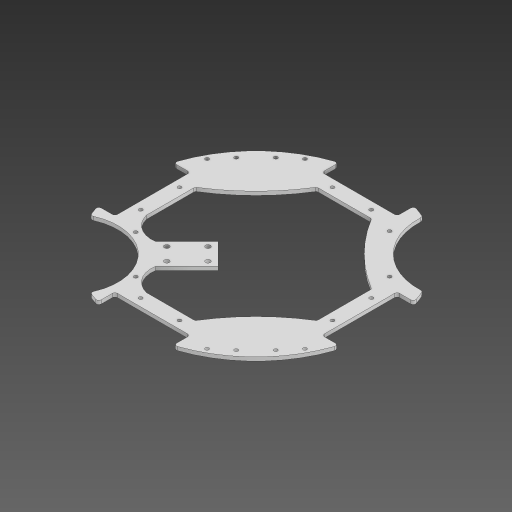
# Autodesk Inventor part: bottom
Saved by Autodesk Inventor 2023 (Build 270158000, 158)
## iProperties
Created: 2025-06-24
Part Number: bottom
Material: Типовые
Document SubType Name: Modeling
Designer: daa
Density: 1 g/cm^3
Appearance: По умолчанию
Author: daa
Autodesk Inventor part; units mm, degrees
ref_plane "YZ Plane" through (0, 0, 0) normal (1, 0, 0) x (0, 1, 0)
ref_plane "XZ Plane" through (0, 0, 0) normal (0, 1, 0) x (-1, 0, 0)
ref_plane "XY Plane" through (0, 0, 0) normal (0, 0, 1) x (1, 0, 0)
sketch "Эскиз1" plane through (0, 0, 0) normal (0, 1, 0) x (-1, 0, 0)
  line L0 (-79, -47.2724) -> (-79, 14.7276)
  line L1 (91.5447, -47.2724) -> (91.5447, 14.7276)
  line L2 (-79, -47.2724) -> (-93, -47.2724)
  line L3 (-79, 14.7276) -> (-93, 14.7276)
  line L4 (91.5447, -47.2724) -> (105.5447, -47.2724)
  line L5 (91.5447, 14.7276) -> (105.5447, 14.7276)
  line L6 (-24.7276, -101.5447) -> (37.2724, -101.5447)
  line L7 (-24.7276, 69) -> (37.2724, 69)
  line L8 (-24.7276, 69) -> (-24.7276, 83)
  line L9 (37.2724, 69) -> (37.2724, 83)
  line L10 (37.2724, -101.5447) -> (37.2724, -115.5447)
  line L11 (-24.7276, -101.5447) -> (-24.7276, -115.5447)
  arc A0 (-93, -47.2724) -> (-24.7276, -115.5447) centre (6.2724, -16.2724) ccw
  arc A1 (105.5447, 14.7276) -> (37.2724, 83) centre (6.2724, -16.2724) ccw
  arc A2 (-24.7276, 83) -> (-93, 14.7276) centre (6.2724, -16.2724) ccw
  arc A3 (37.2724, -115.5447) -> (105.5447, -47.2724) centre (6.2724, -16.2724) ccw
  dimension "d29" = 62
  dimension "d31" = 62
  dimension "d33" = 14
  dimension "d34" = 14
  dimension "d35" = 62
  dimension "d36" = 62
  dimension "d39" = 14
  dimension "d40" = 14
  constraints: 24 end point, 8 point on circle, 4 centre point, 4 horizontal, 3 parallel, 3 vertical, 2 point on line, 1 concentric
  measures "d29" distance of L0.start L0.end
  measures "d31" distance of L1.start L1.end
  measures "d33" distance of L0.end L3.end
  measures "d34" distance of L1.end L5.end
  measures "d35" distance of L6.start L6.end
  measures "d36" distance of L7.start L7.end
  measures "d39" distance of L7.start L8.end
  measures "d40" distance of L6.start L11.end
extrude "motor" add sketch "Эскиз1" along normal blind 3
sketch "Эскиз2" plane through (0, 3, 0) normal (0, 1, 0) x (1, 0, 0)
  arc A0 (24.7276, -83) -> (93, -14.7276) centre (-6.2724, 16.2724) ccw projected
  arc A1 (-37.2724, 115.5447) -> (-105.5447, 47.2724) centre (-6.2724, 16.2724) ccw projected
  circle A2 centre (-6.2724, 16.2724) radius 104
  line L0 (-6.2724, 16.2724) -> (-6.2724, -50.7276)
  arc A3 (-37.2724, 115.5447) -> (-105.5447, 47.2724) centre (-6.2724, 16.2724) ccw projected
  line L1 (-80.4681, -6.5111) -> (-32.5193, -54.4602)
  line L2 (-101.8495, -24.7276) -> (-47.2724, -79.3051)
  arc A4 (-105.5447, -14.7276) -> (-37.2724, -83) centre (-6.2724, 16.2724) ccw projected
  arc A5 (-47.2724, -79.3051) -> (-101.8495, -24.7276) centre (-83.4673, -60.9227) ccw
  arc A6 (24.7276, -83) -> (93, -14.7276) centre (-6.2724, 16.2724) ccw projected
  line L3 (24.3063, 98.7917) -> (72.2554, 50.8426)
  line L4 (35.8032, 111.3809) -> (88.8362, 58.3479)
  arc A7 (93, 47.2724) -> (24.7276, 115.5447) centre (-6.2724, 16.2724) ccw
  arc A8 (35.8032, 111.3809) -> (88.8362, 58.3479) centre (85.4903, 108.035) ccw
  line L5 (-91.5447, -14.7276) -> (-105.5447, -14.7276) projected
  line L6 (-105.5447, -14.7276) -> (-80, -14.7276)
  point P0 (0, 0)
  point P1 (-6.2724, -50.7276)
  point P2 (-101.8495, -24.7276)
  point P3 (-47.2722, -79.3049)
  dimension "d181" = 208
  dimension "d190" = 67
  dimension "d205" = 77.184
  dimension "d207" = 28
  dimension "d208" = 10
  dimension "d214" = 10
  constraints: 12 end point, 7 point on circle, 4 centre point, 2 tangent, 1 point on line, 1 vertical
  measures "d181" diameter of A2
  measures "d190" distance of L0.end L0.start
  measures "d205" distance of L2.start L2.end
  measures "d207" distance between parallel lines of L1 L2
  measures "d208" horizontal distance of A2.end L2.end
  measures "d214" vertical distance of L2.start L5.end
extrude "ball" cut sketch "Эскиз2" against normal blind 3 contours A2 L2 | L2 A5 | L4 A2 | A8 L4
sketch "Эскиз3" plane through (0, 3, 0) normal (0, 1, 0) x (1, 0, 0)
  arc A0 (93, 47.2724) -> (24.7276, 115.5447) centre (-6.2724, 16.2724) ccw projected
  line L0 (-6.2724, 16.2724) -> (97.7276, 16.2724) construction
  line L1 (67.2668, 89.8115) -> (-62.5447, -40)
  circle A1 centre (70.5306, -44.2673) radius 1.5
  circle A2 centre (54.2672, -60.5308) radius 1.5
  circle A3 centre (41.3053, -71.6104) radius 1.5
  circle A4 centre (81.6104, -31.3053) radius 1.5
  arc A5 (24.7276, -83) -> (93, -14.7276) centre (-6.2724, 16.2724) ccw projected
  line L2 (-6.2724, 16.2724) -> (97.7276, 16.2724) construction
  line L3 (-79.8115, 89.8115) -> (67.2668, -57.2668)
  line L4 (-91.5447, 47.2724) -> (-91.5447, -14.7276) projected
  line L5 (-91.5447, 16.2724) -> (79, 16.2724)
  line L6 (24.7276, 101.5447) -> (-37.2724, 101.5447) projected
  line L7 (-6.2724, 101.5447) -> (-6.2724, -69)
  line L8 (-6.2724, 101.5447) -> (-6.2724, -69)
  line L9 (-91.5447, 47.2724) -> (-91.5447, -14.7276) projected
  arc A6 (24.7276, -83) -> (93, -14.7276) centre (-6.2724, 16.2724) ccw projected
  circle A7 centre (-66.812, 93.0753) radius 1.5
  circle A8 centre (-83.0755, 76.8119) radius 1.5
  circle A9 centre (-94.1551, 63.85) radius 1.5
  circle A10 centre (-53.85, 104.1551) radius 1.5
  point P0 (0, 0)
  point P1 (67.2668, -57.2668)
  point P2 (67.2668, -57.2668)
  point P3 (-105.5447, 47.2724)
  point P4 (-79.8115, 89.8115)
  point P5 (-79.8115, 89.8115)
  point P6 (-79.8115, 89.8115)
  dimension "d65" = 3
  dimension "d66" = 3
  dimension "d67" = 3
  dimension "d68" = 3
  dimension "d69" = 23
  dimension "d71" = 57
  dimension "d74" = -12.962
  dimension "d78" = 25.9614
  constraints: 14 end point, 8 centre point, 8 symmetric about line, 4 point on circle, 3 midpoint, 2 horizontal, 2 vertical, 1 point on line, 4 other
  measures "d65" diameter of A1
  measures "d66" diameter of A2
  measures "d67" diameter of A3
  measures "d68" diameter of A4
  measures "d69" distance of A2.centre A1.centre
  measures "d71" distance of A3.centre A4.centre
  measures "d74" vertical distance of A1.centre A4.centre
  measures "d78" vertical distance of A4.centre point (67.267, -57.267)
extrude "hand_mount" cut sketch "Эскиз3" against normal blind 10
sketch "Эскиз4" plane through (0, 3, 0) normal (0, 1, 0) x (1, 0, 0)
  circle A0 centre (-6.2724, 16.2724) radius 104
  arc A1 (-37.2724, 115.5447) -> (-105.5447, 47.2724) centre (-6.2724, 16.2724) ccw projected
  line L0 (-37.2724, -69) -> (24.7276, -69) projected
  line L1 (-79.0447, -1.2276) -> (-79.0447, 38.7724)
  line L2 (-91.5447, 47.2724) -> (-91.5447, -14.7276) projected
  line L3 (-37.2724, -69) -> (24.7276, -69) projected
  line L4 (24.7276, 101.5447) -> (-37.2724, 101.5447) projected
  line L5 (66.5, -6.2276) -> (66.5, 38.7724)
  line L6 (-23.7724, -56.5) -> (16.2276, -56.5)
  line L7 (-28.7724, 89.0447) -> (16.2276, 89.0447)
  arc A2 (16.2276, 89.0447) -> (66.5, 38.7724) centre (144.4083, 166.953) ccw
  arc A3 (66.5, -6.2276) -> (16.2276, -56.5) centre (148.0441, -138.0441) ccw
  arc A4 (-79.0447, 38.7724) -> (-28.7724, 89.0447) centre (-160.5888, 170.5888) ccw
  line L8 (-30.6674, 9.5549) -> (-12.9897, -8.1229)
  line L9 (-12.9897, -8.1229) -> (-38.7992, -33.9322)
  line L10 (-38.7992, -33.9322) -> (-56.4768, -16.2545)
  line L11 (-56.4768, -16.2545) -> (-30.6674, 9.5549)
  circle A5 centre (-31.3151, 1.7173) radius 2
  circle A6 centre (-20.8273, -8.7706) radius 2
  circle A7 centre (-48.273, -15.2405) radius 2
  circle A8 centre (-37.7852, -25.7283) radius 2
  arc A9 (-79.0447, -1.2276) -> (-56.4768, -16.2545) centre (-59.6111, 3.4984) ccw
  arc A10 (-38.7992, -33.9322) -> (-23.7724, -56.5) centre (-19.0463, -37.0664) ccw
  point P0 (0, 0)
  point P1 (-21.8285, 0.716)
  dimension "d84" = 208
  dimension "d101" = 40
  dimension "d102" = 12.5
  dimension "d103" = 8.5
  dimension "d104" = 40
  dimension "d105" = 12.5
  dimension "d106" = 8.5
  dimension "d107" = 150
  dimension "d109" = 155
  dimension "d115" = 155
  dimension "d215" = 25
  dimension "d216" = 36.5
  dimension "d217" = 24.395
  dimension "d218" = 4
  dimension "d219" = 4
  dimension "d220" = 4
  dimension "d221" = 4
  dimension "d222" = 14.832
  dimension "d223" = 10.4878
  dimension "d224" = 6
  dimension "d225" = 5.084
  dimension "d226" = 5.084
  dimension "d227" = 23.982
  dimension "d228" = 23.982
  dimension "d229" = 6
  dimension "d230" = 21.9999
  dimension "d233" = 20
  dimension "d234" = 20
  constraints: 16 end point, 10 centre point, 10 point on circle, 2 parallel, 1 concentric, 1 horizontal, 1 midpoint, 1 perpendicular, 1 vertical
  measures "d84" diameter of A0
  measures "d101" distance of L1.start L1.end
  measures "d102" distance between parallel lines of L2 L1
  measures "d103" vertical distance of L2.start L1.end
  measures "d104" distance of L6.start L6.end
  measures "d105" distance between parallel lines of L6 L0
  measures "d106" horizontal distance of L6.end L0.end
  measures "d107" radius of A2
  measures "d109" radius of A3
  measures "d115" radius of A4
  measures "d215" distance of L9.end L10.end
  measures "d216" distance of L8.end L9.end
  measures "d217" horizontal distance of A0.centre L8.start
  measures "d218" diameter of A5
  measures "d219" diameter of A6
  measures "d220" diameter of A7
  measures "d221" diameter of A8
  measures "d222" distance of A6.centre A5.centre
  measures "d223" horizontal distance of A8.centre A7.centre
  measures "d224" distance from line of L8 A6.centre
  measures "d225" distance from line of L9 A6.centre
  measures "d226" distance from line of L9 A8.centre
  measures "d227" distance of A7.centre A5.centre
  measures "d228" distance of A6.centre A8.centre
  measures "d229" distance from line of L8 A5.centre
  measures "d230" distance of point (-21.829, 0.716) A1.centre
  measures "d233" radius of A9
  measures "d234" radius of A10
extrude "center" cut sketch "Эскиз4" against normal through all contours L1 A4 L7 A2 L5 A3 L6 A10 L9 L8 L11 A9 | A5 | A6 | A7 | A8
sketch "Эскиз6" plane through (0, 3, 0) normal (0, 1, 0) x (1, 0, 0)
  circle A0 centre (-22.2724, 95.2947) radius 1.5
  circle A1 centre (9.7276, 95.2947) radius 1.5
  line L0 (24.7276, 115.5447) -> (24.7276, 101.5447) projected
  line L1 (24.7276, 101.5447) -> (-37.2724, 101.5447) projected
  circle A2 centre (-22.2724, -62.75) radius 1.5
  circle A3 centre (9.7276, -62.75) radius 1.5
  circle A4 centre (-85.2947, 32.2724) radius 1.5
  circle A5 centre (-85.2947, 0.2724) radius 1.5
  circle A6 centre (72.75, 32.2724) radius 1.5
  circle A7 centre (72.75, 0.2724) radius 1.5
  point P0 (0, 0)
  point P1 (24.7276, -69)
  point P2 (-37.2724, -69)
  point P3 (-91.5447, -14.7276)
  point P4 (-91.5447, 47.2724)
  point P5 (79, 47.2724)
  point P6 (79, -14.7276)
  dimension "d135" = 3
  dimension "d136" = 3
  dimension "d137" = 32
  dimension "d138" = 15
  dimension "d139" = 6.25
  dimension "d140" = 3
  dimension "d141" = 3
  dimension "d142" = 6.25
  dimension "d143" = 32
  dimension "d144" = 15
  dimension "d145" = 6.25
  dimension "d146" = 6.25
  dimension "d147" = 3
  dimension "d148" = 3
  dimension "d149" = 32
  dimension "d150" = 15
  dimension "d151" = 6.25
  dimension "d152" = 6.25
  dimension "d153" = 3
  dimension "d154" = 3
  dimension "d155" = 32
  dimension "d156" = 15
  dimension "d157" = 6.25
  dimension "d158" = 6.25
  constraints: 8 centre point
  measures "d135" diameter of A0
  measures "d136" diameter of A1
  measures "d137" distance of A1.centre A0.centre
  measures "d138" distance from line of L0 A1.centre
  measures "d139" distance from line of L1 A1.centre
  measures "d140" diameter of A2
  measures "d141" diameter of A3
  measures "d142" distance from line of L1 A0.centre
  measures "d143" distance of A2.centre A3.centre
  measures "d144" horizontal distance of point (24.728, -69) A3.centre
  measures "d145" vertical distance of point (24.728, -69) A3.centre
  measures "d146" vertical distance of point (-37.272, -69) A2.centre
  measures "d147" diameter of A4
  measures "d148" diameter of A5
  measures "d149" distance of A5.centre A4.centre
  measures "d150" vertical distance of A5.centre point (-91.545, -14.728)
  measures "d151" horizontal distance of A5.centre point (-91.545, -14.728)
  measures "d152" horizontal distance of A4.centre point (-91.545, 47.272)
  measures "d153" diameter of A6
  measures "d154" diameter of A7
  measures "d155" distance of A7.centre A6.centre
  measures "d156" vertical distance of point (79, 47.272) A6.centre
  measures "d157" horizontal distance of point (79, -14.728) A7.centre
  measures "d158" horizontal distance of point (79, 47.272) A6.centre
extrude "Выдавливание6" cut sketch "Эскиз6" against normal blind 10
fillet "Сопряжение1" radius 2 16 edges at (93, 1.5, -47.2724) (24.7276, 1.5, -115.5447) (24.7276, 1.5, -101.5447) (-37.2724, 1.5, -101.5447) (-37.2724, 1.5, -115.5447) (-105.5447, 1.5, -47.2724) (-91.5447, 1.5, -47.2724) (-91.5447, 1.5, 14.7276) (-105.5447, 1.5, 14.7276) (-37.2724, 1.5, 83) (-37.2724, 1.5, 69) (24.7276, 1.5, 69) (24.7276, 1.5, 83) (93, 1.5, 14.7276) (79, 1.5, 14.7276) (79, 1.5, -47.2724)
fillet "Сопряжение2" radius 2 6 edges at (66.5, 1.5, 6.2276) (66.5, 1.5, -38.7724) (16.2276, 1.5, 56.5) (-79.0447, 1.5, -38.7724) (-28.7724, 1.5, -89.0447) (16.2276, 1.5, -89.0447)
fillet "Сопряжение4" radius 2 4 edges at (-101.8495, 1.5, 24.7276) (-47.2722, 1.5, 79.3049) (35.8032, 1.5, -111.3809) (88.8362, 1.5, -58.3479)
sketch "Эскиз8" plane through (0, 3, 0) normal (0, 1, 0) x (1, 0, 0)
  circle A0 centre (-71.3475, -17.7584) radius 1.5
  circle A1 centre (-39.5277, -49.5782) radius 1.5
  line L0 (-71.3475, -17.7584) -> (-39.5277, -49.5782)
  line L1 (-71.3475, -17.7584) -> (-26.3475, -17.7584) construction
  arc A2 (-46.39, -77.4532) -> (-99.9979, -23.8454) centre (-83.4673, -60.9227) ccw projected
  line L2 (-54.3769, -32.6076) -> (-55.4376, -33.6683)
  line L3 (-54.3769, -32.6076) -> (-52.8769, -32.6076) construction
  point P0 (0, 0)
  dimension "d235" = 3
  dimension "d236" = 3
  dimension "d237" = 45
  dimension "d238" = 45
  dimension "d239" = 1.5
  dimension "d240" = 135
  constraints: 8 end point, 2 centre point, 2 equal length, 2 horizontal, 1 coincident, 1 midpoint, 1 point on circle
  measures "d235" diameter of A0
  measures "d236" diameter of A1
  measures "d237" distance of L0.start L0.end
  measures "d238" angle of L0 L1
  measures "d239" distance of L2.end L2.start
  measures "d240" angle of L2 L3
extrude "Выдавливание7" cut sketch "Эскиз8" against normal through all contours A0 | A1
sketch "Эскиз9" plane through (0, 3, 0) normal (0, 1, 0) x (1, 0, 0)
  circle A0 centre (32.4965, 87.5681) radius 1.5
  circle A1 centre (65.0234, 55.0412) radius 1.5
  line L0 (32.4965, 87.5681) -> (65.0234, 55.0412)
  line L1 (32.4965, 87.5681) -> (78.4965, 87.5681) construction
  arc A2 (35.7303, 110.0204) -> (87.4757, 58.275) centre (85.4903, 108.035) ccw projected
  line L2 (50.2767, 72.8214) -> (66.5401, 56.5579)
  line L3 (50.2767, 72.8214) -> (73.2767, 72.8214) construction
  line L4 (50.2767, 72.8214) -> (48.7599, 71.3046)
  line L5 (50.2767, 72.8214) -> (52.4217, 72.8214) construction
  point P0 (0, 0)
  dimension "d243" = 3
  dimension "d244" = 3
  dimension "d245" = 46
  dimension "d246" = 45
  dimension "d247" = 23
  dimension "d248" = 45
  dimension "d250" = 2.145
  dimension "d251" = 135
  constraints: 12 end point, 3 equal length, 3 horizontal, 2 centre point, 1 coincident, 1 midpoint, 1 point on circle
  measures "d243" diameter of A0
  measures "d244" diameter of A1
  measures "d245" distance of L0.start L0.end
  measures "d246" angle of L0 L1
  measures "d247" distance of L2.start L2.end
  measures "d248" angle of L2 L3
  measures "d250" distance of L4.end L2.start
  measures "d251" angle of L4 L5
extrude "Выдавливание8" cut sketch "Эскиз9" against normal through all
